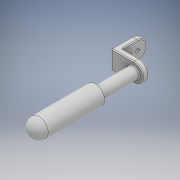
# Autodesk Inventor part: toe
Saved by Autodesk Inventor 2018 (Build 220112000, 112)
## iProperties
Created: 2018-04-27
Part Number: toe
Material: Generic
Document SubType Name: Modeling
Designer: Matyi
Density: 1 g/cm^3
Appearance: Default
Author: Matyi
Autodesk Inventor part; units mm, degrees
ref_plane "YZ Plane" through (0, 0, 0) normal (1, 0, 0) x (0, 1, 0)
ref_plane "XZ Plane" through (0, 0, 0) normal (0, 1, 0) x (-1, 0, 0)
ref_plane "XY Plane" through (0, 0, 0) normal (0, 0, 1) x (1, 0, 0)
sketch "Sketch2" plane through (0, 0, 0) normal (0, 1, 0) x (-1, 0, 0)
  line L0 (0, 0) -> (17, 0)
  line L1 (17, 0) -> (17, -10)
  line L2 (17, -10) -> (0, -10)
  line L3 (0, -10) -> (0, 0)
  line L4 (17, 0) -> (14, 0)
  line L5 (14, -10) -> (17, -10)
  line L6 (17, -10) -> (17, 0)
  dimension "d2" = 17
  dimension "d3" = 10
  constraints: 14 end point, 3 parallel, 2 horizontal, 1 perpendicular, 1 point on line
  measures "d2" distance of L1.end L2.end
  measures "d3" distance of L0.end L1.end
extrude "Extrusion1" add sketch "Sketch2" along normal blind 3
fillet "Fillet1" radius 5 2 edges at (0, 1.5, -10) (0, 1.5, 0)
sketch "Sketch5" plane through (0, 0, 0) normal (0, -1, 0) x (1, 0, 0)
  circle A0 centre (-5, -5) radius 3
  line L0 (-17, 0) -> (-5, 0) projected
  arc A1 (-5, -10) -> (-5, 0) centre (-5, -5) ccw projected
  point P0 (0, 0)
  dimension "d19" = 6
  dimension "d20" = 5
  dimension "d21" = 0
  constraints: 1 centre point
  measures "d19" diameter of A0
  measures "d20" distance from line of L0 A0.centre
  measures "d21" distance of A1.centre A0.centre
extrude "Extrusion4" add sketch "Sketch5" along normal blind 20
sketch "Sketch6" plane through (-5, -20, -5) normal (0, -1, 0) x (1, 0, 0)
  circle A0 centre (0, 0) radius 5
  point P0 (5, 5)
  dimension "d24" = 10
  constraints: 1 centre point
  measures "d24" diameter of A0
extrude "Extrusion5" add sketch "Sketch6" along normal blind 35.6
fillet "Fillet2" radius 5 1 edges at (-10, -55.6, -5)
sketch "Sketch7" plane through (0, 3, 0) normal (0, 1, 0) x (1, 0, 0)
  line L0 (-17, 0) -> (-17, 10) projected
  line L1 (-17, 0) -> (-14, 0)
  line L2 (-14, 0) -> (-14, 10)
  line L3 (-14, 10) -> (-17, 10)
  line L4 (-17, 10) -> (-17, 0)
  point P0 (0, 0)
  dimension "d29" = 3
  dimension "d30" = 10
  constraints: 8 end point, 2 parallel, 1 horizontal, 1 perpendicular
  measures "d29" distance of L3.end L2.end
  measures "d30" distance of L2.end L1.end
extrude "Extrusion6" add sketch "Sketch7" along normal blind 13
fillet "Fillet4" radius 5 2 edges at (-15.5, 16, 0) (-15.5, 16, -10)
sketch "Sketch8" plane through (-14, 3, 0) normal (1, 0, 0) x (0, 0, -1)
  circle A0 centre (5, 8) radius 1
  circle A1 centre (5, 4) radius 1
  arc A2 (10, 8) -> (0, 8) centre (5, 8) ccw projected
  line L0 (0, 0) -> (0, 8) projected
  line L1 (10, 0) -> (10, 8) projected
  point P0 (0, -3)
  dimension "d34" = 2
  dimension "d35" = 2
  dimension "d36" = 0
  dimension "d37" = 4
  dimension "d38" = 5
  dimension "d39" = 5
  dimension "d40" = 10
  dimension "d41" = 5
  constraints: 2 centre point
  measures "d34" diameter of A0
  measures "d35" diameter of A1
  measures "d36" distance of A2.centre A0.centre
  measures "d37" distance of A1.centre A0.centre
  measures "d38" distance from line of L0 A1.centre
  measures "d39" distance from line of L1 A0.centre
  measures "d40" distance between parallel lines of L1 L0
  measures "d41" distance from line of L0 A0.centre
extrude "Extrusion7" cut sketch "Sketch8" against normal blind 3
fillet "Fillet5" radius 0.5 17 edges at (-10, -20, -5) (-8, -20, -5) (-11, 0, -10) (-11, 0, 0) (-1.4644, 0, -8.5356) (-8, 0, -5) (-9.5, 3, 0) (-9.5, 3, -10) (-1.4644, 3, -8.5356) (-14, 3, -5) (-14, 14.5356, -1.4644) (-14, 7, 0) (-14, 7, -10) (-17, 5.5, 0) (-17, 5.5, -10) (-17, 14.5356, -1.4644) (-17, 0, -5)
body "Solid1"
